rod_label_clip (Autodesk Fusion 360 design; units mm, degrees)
part number: 2026-09-05-07-00-16-324
Autodesk Fusion 360 part; units mm, degrees
sketch "Ring" plane through (0, 0, 0) normal (0, 1, 0) x (1, 0, 0)
  circle A0 centre (0, 0) radius 17.05
  circle A1 centre (0, 0) radius 19.45
  dimension "d124" = 34.1
  dimension "d125" = 38.9
  constraint coincident A0.centre A1.centre
  constraint concentric A0 A1
  measures "d124" diameter of A0
  measures "d125" diameter of A1
extrude "Ring (1)" add sketch "Ring" along normal mid plane 9
sketch "Mouth" plane through (0, 0, 0) normal (0, 1, 0) x (1, 0, 0)
  line L0 (0, 0) -> (42.3486, -24.45)
  line L1 (42.3486, -24.45) -> (0, -48.9)
  line L2 (0, -48.9) -> (-42.3486, -24.45)
  line L3 (-42.3486, -24.45) -> (0, 0)
  line L4 (0, 0) -> (0, -48.9) construction
  dimension "d128" = 48.9
  dimension "d129" = 48.9
  dimension "d130" = 48.9
  dimension "d131" = 60
  dimension "d132" = 60
  constraint coincident L0.start L3.end
  constraint vertical L4
  constraint coincident L1.end L2.start
  measures "d128" distance of L0.start L0.end
  measures "d129" distance of L0.start L2.end
  measures "d130" distance of L0.start L1.end
  measures "d131" angle of L0 L4
  measures "d132" angle of L3 L4
extrude "Mouth (1)" cut sketch "Mouth" along normal mid plane 19
sketch "Stem" plane through (0, 0, 0) normal (0, 1, 0) x (1, 0, 0)
  line L0 (12.6501, 13.209) -> (20.8135, 22.9377)
  line L1 (20.8135, 22.9377) -> (18.975, 24.4804)
  line L2 (18.975, 24.4804) -> (10.8116, 14.7517)
  line L3 (10.8116, 14.7517) -> (12.6501, 13.209)
  dimension "d135" = 12.6501
  dimension "d136" = 13.209
  dimension "d137" = 20.8135
  dimension "d138" = 22.9377
  dimension "d139" = 18.975
  dimension "d140" = 24.4804
  dimension "d141" = 10.8116
  dimension "d142" = 14.7517
  measures "d135" horizontal distance of origin L0.start
  measures "d136" vertical distance of origin L0.start
  measures "d137" horizontal distance of origin L0.end
  measures "d138" vertical distance of origin L0.end
  measures "d139" horizontal distance of origin L1.end
  measures "d140" vertical distance of origin L1.end
  measures "d141" horizontal distance of origin L2.end
  measures "d142" vertical distance of origin L2.end
extrude "Stem (1)" add sketch "Stem" along normal mid plane 9
sketch "Label face" plane through (0, 0, 0) normal (0, 1, 0) x (1, 0, 0)
  line L0 (20.8135, 22.9377) -> (39.4544, 45.153)
  line L1 (39.4544, 45.153) -> (37.6159, 46.6957)
  line L2 (37.6159, 46.6957) -> (18.975, 24.4804)
  line L3 (18.975, 24.4804) -> (20.8135, 22.9377)
  dimension "d145" = 20.8135
  dimension "d146" = 22.9377
  dimension "d147" = 39.4544
  dimension "d148" = 45.153
  dimension "d149" = 37.6159
  dimension "d150" = 46.6957
  dimension "d151" = 18.975
  dimension "d152" = 24.4804
  measures "d145" horizontal distance of origin L0.start
  measures "d146" vertical distance of origin L0.start
  measures "d147" horizontal distance of origin L0.end
  measures "d148" vertical distance of origin L0.end
  measures "d149" horizontal distance of origin L1.end
  measures "d150" vertical distance of origin L1.end
  measures "d151" horizontal distance of origin L2.end
  measures "d152" vertical distance of origin L2.end
extrude "Label face (1)" add sketch "Label face" along normal mid plane 58
equation "clipWidth = 9.0 mm" comment "ring and stem width along the rod"
equation "faceWidth = 58.0 mm" comment "label face width along the rod"
equation "rodOuterDiameter = 33.4 mm" comment "rod the clip snaps onto"
equation "clipClearance = 0.7 mm" comment "diametral, so the clip slides"
equation "clipWall = 2.4 mm" comment "ring wall thickness"
equation "mouthHalfAngleDeg = 60.0 deg" comment "half the mouth opening"
equation "paddleThickness = 2.4 mm" comment "stem and label face thickness"
equation "stemEndRadius = ( rodOuterDiameter + clipClearance + 2 * clipWall ) / 2 + stemLength" comment "derived: stem ends, label face begins"
equation "faceEndRadius = stemEndRadius + faceHeight" comment "derived: outer edge of the label face"
equation "paddleAngleDeg = 50.0 deg" comment "paddle drop below horizontal"
equation "stemStartRadius = ( rodOuterDiameter + clipClearance ) / 2 + clipWall / 2" comment "derived: stem starts mid ring wall"
equation "stemLength = 11.5 mm" comment "stem reach beyond the ring outer wall"
equation "faceHeight = 29.0 mm" comment "label face, from stem end outward"
equation "d124 = rodOuterDiameter + clipClearance"
equation "d125 = rodOuterDiameter + clipClearance + 2 * clipWall"
equation "d126 = clipWidth"
equation "d128 = ( ( rodOuterDiameter + clipClearance + 2 * clipWall ) / 2 + 5 mm ) / cos(mouthHalfAngleDeg)"
equation "d129 = ( ( rodOuterDiameter + clipClearance + 2 * clipWall ) / 2 + 5 mm ) / cos(mouthHalfAngleDeg)"
equation "d130 = ( ( rodOuterDiameter + clipClearance + 2 * clipWall ) / 2 + 5 mm ) / cos(mouthHalfAngleDeg)"
equation "d131 = mouthHalfAngleDeg"
equation "d132 = mouthHalfAngleDeg"
equation "d133 = clipWidth + 10 mm"
equation "d135 = stemStartRadius * cos(paddleAngleDeg) + paddleThickness / 2 * sin(paddleAngleDeg)"
equation "d136 = stemStartRadius * sin(paddleAngleDeg) - paddleThickness / 2 * cos(paddleAngleDeg)"
equation "d137 = stemEndRadius * cos(paddleAngleDeg) + paddleThickness / 2 * sin(paddleAngleDeg)"
equation "d138 = stemEndRadius * sin(paddleAngleDeg) - paddleThickness / 2 * cos(paddleAngleDeg)"
equation "d139 = stemEndRadius * cos(paddleAngleDeg) - paddleThickness / 2 * sin(paddleAngleDeg)"
equation "d140 = stemEndRadius * sin(paddleAngleDeg) + paddleThickness / 2 * cos(paddleAngleDeg)"
equation "d141 = stemStartRadius * cos(paddleAngleDeg) - paddleThickness / 2 * sin(paddleAngleDeg)"
equation "d142 = stemStartRadius * sin(paddleAngleDeg) + paddleThickness / 2 * cos(paddleAngleDeg)"
equation "d143 = clipWidth"
equation "d145 = stemEndRadius * cos(paddleAngleDeg) + paddleThickness / 2 * sin(paddleAngleDeg)"
equation "d146 = stemEndRadius * sin(paddleAngleDeg) - paddleThickness / 2 * cos(paddleAngleDeg)"
equation "d147 = faceEndRadius * cos(paddleAngleDeg) + paddleThickness / 2 * sin(paddleAngleDeg)"
equation "d148 = faceEndRadius * sin(paddleAngleDeg) - paddleThickness / 2 * cos(paddleAngleDeg)"
equation "d149 = faceEndRadius * cos(paddleAngleDeg) - paddleThickness / 2 * sin(paddleAngleDeg)"
equation "d150 = faceEndRadius * sin(paddleAngleDeg) + paddleThickness / 2 * cos(paddleAngleDeg)"
equation "d151 = stemEndRadius * cos(paddleAngleDeg) - paddleThickness / 2 * sin(paddleAngleDeg)"
equation "d152 = stemEndRadius * sin(paddleAngleDeg) + paddleThickness / 2 * cos(paddleAngleDeg)"
equation "d153 = faceWidth"
named bodies: "rod_label_clip"
